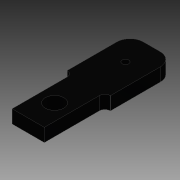
# Autodesk Inventor part: Fixture_Airpot_Support
Saved by Autodesk Inventor 2015 (Build 190159000, 159)
## iProperties
Created: 2014-12-16
Part Number: Fixture_Airpot_Support
Material: Generic
Document SubType Name: Modeling
Designer: amarschn
Density: 1 g/cm^3
Appearance: Anodized - Black
Author: amarschn
Autodesk Inventor part; units mm, degrees
ref_plane "YZ Plane" through (0, 0, 0) normal (1, 0, 0) x (0, 1, 0)
ref_plane "XZ Plane" through (0, 0, 0) normal (0, 1, 0) x (-1, 0, 0)
ref_plane "XY Plane" through (0, 0, 0) normal (0, 0, 1) x (1, 0, 0)
sketch "Sketch1" plane through (0, 0, 0) normal (0, 1, 0) x (-1, 0, 0)
  line L0 (15.5575, -24.13) -> (15.5575, 29.21)
  line L1 (15.5575, 29.21) -> (-15.5575, 29.21)
  line L2 (-15.5575, 29.21) -> (-15.5575, -24.13)
  line L3 (-15.5575, -29.21) -> (15.5575, 29.21) construction
  line L4 (15.5575, -29.21) -> (-15.5575, 29.21) construction
  line L5 (20.6375, -29.21) -> (20.955, -29.21)
  line L6 (20.955, -29.21) -> (20.955, -77.47)
  line L7 (8.255, -90.17) -> (-8.255, -90.17)
  line L8 (-20.955, -77.47) -> (-20.955, -29.21)
  line L9 (-20.955, -29.21) -> (-20.6375, -29.21)
  arc A0 (15.5575, -24.13) -> (20.6375, -29.21) centre (20.6375, -24.13) ccw
  arc A1 (-20.6375, -29.21) -> (-15.5575, -24.13) centre (-20.6375, -24.13) ccw
  circle A2 centre (0, 3.81) radius 8.89
  arc A3 (8.255, -90.17) -> (20.955, -77.47) centre (8.255, -77.47) ccw
  arc A4 (-20.955, -77.47) -> (-8.255, -90.17) centre (-8.255, -77.47) ccw
  point P0 (0, 0)
  point P1 (20.955, -90.17)
  point P2 (-20.955, -90.17)
  dimension "d0" = 5.08
  dimension "d1" = 31.115
  dimension "d2" = 41.91
  dimension "d3" = 60.96
  dimension "d4" = 119.38
  dimension "d5" = 17.78
  dimension "d6" = 25.4
  dimension "d7" = 12.7
  constraints: 20 end point, 9 point on line, 8 point on circle, 8 tangent, 5 centre point, 4 perpendicular, 2 equal radius, 2 midpoint, 1 collinear, 1 horizontal, 1 parallel
  measures "d0" radius of A0
  measures "d1" distance of L0.end L1.end
  measures "d2" distance of point (20.955, -90.17) point (-20.955, -90.17)
  measures "d3" distance of L5.end point (20.955, -90.17)
  measures "d4" distance between parallel lines of L7 L1
  measures "d5" diameter of A2
  measures "d6" distance from line of L1 A2.centre
  measures "d7" radius of A3
extrude "Extrusion1" add sketch "Sketch1" along normal blind 12.7
sketch "Sketch2" plane through (0, 12.7, 0) normal (0, 1, 0) x (1, 0, 0)
  line L0 (-8.255, 90.17) -> (8.255, 90.17) projected
  point P0 (0, 0)
  point P1 (0, 64.77)
  dimension "d19" = 25.4
  measures "d19" distance from line of L0 point (0, 64.77)
hole "Hole2" at (0, 12.7, -64.77) direction (0, -1, 0) diameter 6.35 end through all
body "Solid1"
